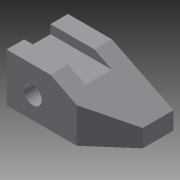
# Autodesk Inventor part: HW 5 Part 3
Saved by Autodesk Inventor 2015 (Build 190159000, 159)
## iProperties
Created: 2016-02-03
Part Number: HW 5 Part 3
Material: Generic
Document SubType Name: Modeling
Designer: melissa.roth
Density: 1 g/cm^3
Appearance: Default
Author: melissa.roth
Autodesk Inventor part; units mm, degrees
ref_plane "YZ Plane" through (0, 0, 0) normal (1, 0, 0) x (0, 1, 0)
ref_plane "XZ Plane" through (0, 0, 0) normal (0, 1, 0) x (-1, 0, 0)
ref_plane "XY Plane" through (0, 0, 0) normal (0, 0, 1) x (1, 0, 0)
sketch "Sketch1" plane through (0, 0, 0) normal (0, 0, 1) x (1, 0, 0)
  line L0 (0, 0) -> (0, 69.85)
  line L1 (0, 69.85) -> (63.5, 69.85)
  line L2 (152.4, 0) -> (0, 0)
  line L3 (63.5, 69.85) -> (152.4, 25.4)
  line L4 (152.4, 25.4) -> (152.4, 0)
  circle A0 centre (38.1, 31.75) radius 12.7
  dimension "d0" = 69.85
  dimension "d1" = 152.4
  dimension "d2" = 63.5
  dimension "d3" = 25.4
  dimension "d4" = 25.4
  dimension "d5" = 38.1
  dimension "d6" = 31.75
  constraints: 10 end point, 1 centre point, 1 parallel, 1 vertical
  measures "d0" distance of L0.start L0.end
  measures "d1" distance of L2.start L0.start
  measures "d2" distance of L0.end L1.end
  measures "d3" distance of L3.end L2.start
  measures "d4" diameter of A0
  measures "d5" distance from line of L0 A0.centre
  measures "d6" distance from line of L2 A0.centre
extrude "Extrusion1" add sketch "Sketch1" along normal blind 88.9
sketch "Sketch2" plane through (0, 0, 0) normal (0, -1, 0) x (1, 0, 0)
  line L0 (152.4, 88.9) -> (152.4, 44.45)
  line L1 (152.4, 0) -> (152.4, 88.9) projected
  line L2 (152.4, 44.45) -> (152.4, 0)
  line L3 (0, 88.9) -> (101.6, 88.9)
  line L4 (0, 88.9) -> (152.4, 88.9) projected
  line L5 (101.6, 88.9) -> (152.4, 44.45)
  line L6 (101.6, 88.9) -> (152.4, 88.9)
  point P0 (0, 0)
  dimension "d9" = 44.45
  dimension "d11" = 101.6
  constraints: 10 end point, 2 collinear, 1 midpoint, 1 point on line
  measures "d9" distance of L0.start L0.end
  measures "d11" distance of L3.start L3.end
extrude "Extrusion2" cut sketch "Sketch2" against normal blind 88.9
sketch "Sketch3" plane through (0, 69.85, 0) normal (0, 1, 0) x (1, 0, 0)
  line L0 (0, 0) -> (0, -88.9) projected
  line L1 (0, -63.5) -> (107.2114, -63.5)
  line L2 (107.2114, -63.5) -> (107.2114, -25.4)
  line L3 (107.2114, -25.4) -> (0, -25.4)
  line L4 (0, -25.4) -> (0, -63.5)
  dimension "d14" = 25.4
  dimension "d15" = 25.4
  constraints: 8 end point, 2 parallel, 1 horizontal, 1 perpendicular, 1 point on line
  measures "d14" distance of L0.end L1.start
  measures "d15" distance of L0.start L3.end
extrude "Extrusion3" cut sketch "Sketch3" against normal blind 12.7
equation "\"d0\" = 2.75 * d3"
equation "\"d5\" = 0.25 * d1"
equation "\"d6\" = 1.25 * d3"
body "Solid1"
